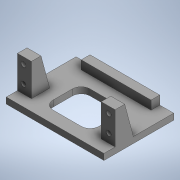
# Autodesk Inventor part: MG996R Attachment Test
Saved by Autodesk Inventor 2020.5 (Build 245400000, 400)
## iProperties
Created: 2023-03-16
Part Number: MG996R Attachment Test
Material: Generic
Document SubType Name: Modeling
Designer: Wes
Density: 1 g/cm^3
Appearance: Default
Author: Wes
Autodesk Inventor part; units mm, degrees
ref_plane "YZ Plane" through (0, 0, 0) normal (1, 0, 0) x (0, 1, 0)
ref_plane "XZ Plane" through (0, 0, 0) normal (0, 1, 0) x (-1, 0, 0)
ref_plane "XY Plane" through (0, 0, 0) normal (0, 0, 1) x (1, 0, 0)
sketch "Base" plane through (0, 0, 0) normal (0, 0, 1) x (1, 0, 0)
  line L0 (0, 0) -> (-40, 0)
  line L1 (-40, 0) -> (-40, 56)
  line L2 (-40, 56) -> (0, 56)
  line L3 (0, 56) -> (0, 0)
  dimension "d0" = 40
  dimension "d1" = 56
  constraints: 8 end point, 2 parallel, 1 horizontal, 1 perpendicular
  measures "d0" distance of L1.end L2.end
  measures "d1" distance of L0.end L1.end
extrude "Extrusion1" add sketch "Base" along normal mid plane 3.5
sketch "Backstop" plane through (0, 0, 1.75) normal (0, 0, 1) x (1, 0, 0)
  line L0 (-40, 28) -> (-40, 8)
  line L1 (-40, 28) -> (-40, 48)
  line L2 (-40, 8) -> (-35, 8)
  line L3 (-35, 8) -> (-35, 48)
  line L4 (-35, 48) -> (-40, 48)
  point P0 (0, 0)
  dimension "d6" = 40
  dimension "d7" = 5
  constraints: 10 end point, 1 horizontal, 1 perpendicular, 1 vertical
  measures "d6" distance of L1.end L0.end
  measures "d7" distance of L0.end L2.end
extrude "Extrusion2" add sketch "Backstop" along normal blind 5
sketch "Attachment Towers" plane through (0, 0, 1.75) normal (0, 0, 1) x (1, 0, 0)
  line L0 (-40, 8) -> (-35, 8) construction
  line L1 (-35, 8) -> (-6.4, 8) construction
  line L2 (-35, 48) -> (-40, 48) construction
  line L3 (-35, 48) -> (-6.4, 48) construction
  line L4 (-6.4, 8) -> (-11.9, 8)
  line L5 (-11.9, 8) -> (-11.9, 0)
  line L6 (-11.9, 0) -> (-6.4, 0)
  line L7 (-6.4, 0) -> (-6.4, 8)
  line L8 (-6.4, 48) -> (-11.9, 48)
  line L9 (-11.9, 48) -> (-11.9, 56)
  line L10 (-11.9, 56) -> (-6.4, 56)
  line L11 (-6.4, 56) -> (-6.4, 48)
  point P0 (0, 0)
  dimension "d10" = 28.6
  dimension "d11" = 5.5
  dimension "d12" = 8
  constraints: 20 end point, 4 horizontal, 4 parallel, 2 perpendicular
  measures "d10" distance of L0.end L1.end
  measures "d11" distance of L6.end L5.end
  measures "d12" distance of L5.end L4.end
extrude "Extrusion3" add sketch "Attachment Towers" along normal blind 18.5
sketch "Screw Holes" plane through (-6.4, 0, 1.75) normal (1, 0, 0) x (0, 0, -1)
  line L0 (0, 48) -> (0, 50.3) construction
  line L1 (0, 50.3) -> (-7.15, 50.3) construction
  circle A0 centre (-5.025, 52.425) radius 2.125 construction
  line L2 (-7.15, 50.3) -> (-7.15, 59.5367) construction
  line L3 (-2.9, 52.425) -> (-16.97, 52.425) construction
  circle A1 centre (-14.845, 52.425) radius 2.125 construction
  line L4 (-16.97, 50.3) -> (-16.97, 59.5367) construction
  circle A2 centre (-14.845, 52.425) radius 1.4
  circle A3 centre (-5.025, 52.425) radius 1.4
  line L5 (0, 48) -> (0, 8) construction
  line L6 (0, 28) -> (-23.658, 28) construction
  circle A4 centre (-14.845, 3.575) radius 1.4
  circle A5 centre (-5.025, 3.575) radius 1.4
  point P0 (1.75, 0)
  dimension "d18" = 4.25
  dimension "d15" = 2.3
  dimension "d16" = 7.15
  dimension "d20" = 14.07
  dimension "d21" = 4.25
  dimension "d22" = 2.8
  dimension "d23" = 2.8
  constraints: 12 end point, 5 centre point, 3 horizontal, 2 coincident, 2 point on line, 2 symmetric about line, 2 vertical, 1 horizontal alignment, 1 midpoint, 1 parallel, 1 tangent, 4 other
  measures "d15" distance of L0.start L0.end
  measures "d16" distance of L0.end L1.end
  measures "d20" distance of L3.start L3.end
  measures "d21" diameter of A1
  measures "d22" diameter of A2
  measures "d23" diameter of A3
extrude "Extrusion4" cut sketch "Screw Holes" against normal blind 4
draft "FaceDraft1" angle 15 pull direction (0, 0, 1) faces at (-11.9, 5.3333, 7.9167) (-11.9, 53.3333, 7.9167) fixed edges at (-11.9, 4, 20.25) (-11.9, 52, 20.25)
sketch "Sketch5" plane through (0, 0, 1.75) normal (0, 0, 1) x (1, 0, 0)
  line L0 (-35, 48) -> (-35, 8) construction
  line L1 (-35, 28) -> (0, 28) construction
  line L2 (-11.9296, 14.8954) -> (-23.0704, 14.8954)
  line L3 (-28.0704, 19.8954) -> (-28.0704, 36.1046)
  line L4 (-23.0704, 41.1046) -> (-11.9296, 41.1046)
  line L5 (-6.9296, 36.1046) -> (-6.9296, 19.8954)
  line L6 (-6.9296, 14.8954) -> (-28.0704, 41.1046) construction
  line L7 (-28.0704, 14.8954) -> (-6.9296, 41.1046) construction
  arc A0 (-11.9296, 14.8954) -> (-6.9296, 19.8954) centre (-11.9296, 19.8954) ccw
  arc A1 (-28.0704, 19.8954) -> (-23.0704, 14.8954) centre (-23.0704, 19.8954) ccw
  arc A2 (-23.0704, 41.1046) -> (-28.0704, 36.1046) centre (-23.0704, 36.1046) ccw
  arc A3 (-6.9296, 36.1046) -> (-11.9296, 41.1046) centre (-11.9296, 36.1046) ccw
  point P0 (-17.5, 28)
  dimension "d27" = 5
  dimension "d28" = 5
  constraints: 14 end point, 8 point on circle, 8 point on line, 8 tangent, 4 centre point, 4 midpoint, 2 equal radius, 2 parallel, 1 horizontal, 1 perpendicular
  measures "d27" radius of A0
  measures "d28" radius of A3
extrude "Extrusion5" cut sketch "Sketch5" against normal through all
body "Solid1"
